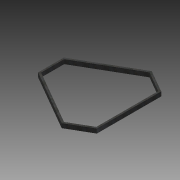
# Autodesk Inventor part: BasePlatform
Saved by Autodesk Inventor 2015 SP1 (Build 190203100, 203)
## iProperties
Created: 2016-02-02
Part Number: BasePlatform
Material: Steel
Document SubType Name: Modeling
Designer: tuttlem
Mass: 32237.8 g
Surface Area: 4761.07 cm^2
Volume: 4106.72 cm^3
Density: 7.85 g/cm^3
Appearance: Plate
Author: tuttlem
Autodesk Inventor part; units mm, degrees
ref_plane "YZ Plane" through (0, 0, 0) normal (1, 0, 0) x (0, 1, 0)
ref_plane "XZ Plane" through (0, 0, 0) normal (0, 1, 0) x (-1, 0, 0)
ref_plane "XY Plane" through (0, 0, 0) normal (0, 0, 1) x (1, 0, 0)
sketch "Sketch1" plane through (0, 0, 0) normal (0, 1, 0) x (-1, 0, 0)
  line L0 (908.9386, 54.09) -> (249.0272, 435.09)
  line L1 (-14.9373, 282.69) -> (-14.9373, -479.31)
  line L2 (249.0272, -631.71) -> (908.9386, -250.71)
  line L3 (908.9386, 54.09) -> (908.9386, -250.71)
  line L4 (249.0272, 435.09) -> (-14.9373, 282.69)
  line L5 (249.0272, -631.71) -> (-14.9373, -479.31)
  line L6 (890.6147, 37.6652) -> (248.5173, 408.3803)
  line L7 (248.5173, 408.3803) -> (5.5839, 268.1226)
  line L8 (5.5839, 268.1226) -> (5.5839, -465.0826)
  line L9 (5.5839, -465.0826) -> (249.9104, -606.1446)
  line L10 (249.9104, -606.1446) -> (890.6147, -236.2337)
  line L11 (890.6147, -236.2337) -> (890.6147, 37.6652)
  point P0 (585.2718, 213.955)
  point P1 (585.2718, -412.5235)
  point P2 (549.3078, 234.7189)
  point P3 (5.5839, -79.2003)
  point P4 (550.9952, -432.3131)
  point P5 (5.5839, -117.4198)
  point P6 (522.9199, 249.9539)
  point P7 (5.5839, -48.7302)
  point P8 (5.5839, -143.4951)
  point P9 (528.4133, -445.3508)
  point P10 (612.3851, 198.3012)
  point P11 (612.3851, -396.8697)
  dimension "d47" = 22.5819
  constraints: 24 end point, 12 point on line, 6 parallel
  measures "d47" distance between parallel lines of L9 L5
extrude "Extrusion6" add sketch "Sketch1" along normal blind 50.8
body "Solid3"
